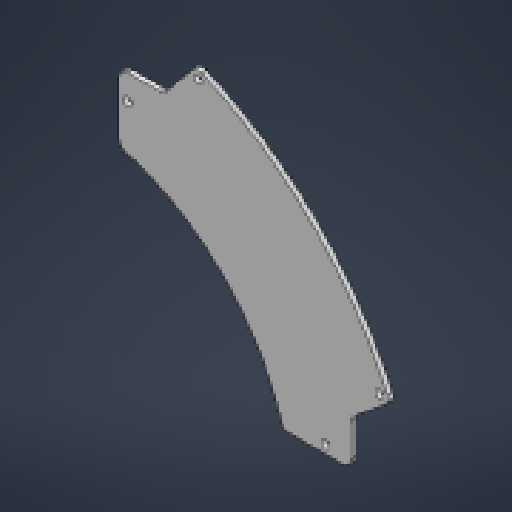
# Autodesk Inventor part: MotorDriver_PCB
Saved by Autodesk Inventor 2024.2 (Build 282272000, 272)
## iProperties
Created: 2023-12-22
Part Number: MotorDriver_PCB
Material: 一般
Document SubType Name: Modeling
Designer: Hanaoka
Density: 1 g/cm^3
Appearance: 既定
Author: Hanaoka
Autodesk Inventor part; units mm, degrees
ref_plane "YZ Plane" through (0, 0, 0) normal (1, 0, 0) x (0, 1, 0)
ref_plane "XZ Plane" through (0, 0, 0) normal (0, 1, 0) x (-1, 0, 0)
ref_plane "XY Plane" through (0, 0, 0) normal (0, 0, 1) x (1, 0, 0)
sketch "スケッチ1" plane through (0, 0, 0) normal (0, 0, 1) x (1, 0, 0)
  line L0 (54, -47.9205) -> (54, -40.1498) projected
  arc A0 (54.7258, -38.6082) -> (54, -40.1498) centre (56, -40.1498) ccw projected
  line L1 (54.7258, -38.6082) -> (62.3004, -32.3475) projected
  arc A1 (62.3004, -32.3475) -> (62.8611, -30.0103) centre (61.0262, -30.8059) ccw projected
  arc A2 (62.8611, -30.0103) -> (17.9102, 14.9406) centre (-16.5, -64.4205) ccw projected
  arc A3 (17.9102, 14.9406) -> (15.573, 14.3799) centre (17.1146, 13.1057) ccw projected
  line L2 (15.573, 14.3799) -> (9.3123, 6.8053) projected
  arc A4 (7.7707, 6.0795) -> (9.3123, 6.8053) centre (7.7707, 8.0795) ccw projected
  line L3 (7.7707, 6.0795) -> (0, 6.0795) projected
  arc A5 (0, 6.0795) -> (-2, 4.0795) centre (0, 4.0795) ccw projected
  line L4 (-2, 4.0795) -> (-2, -8.817) projected
  arc A6 (-2, -8.817) -> (-0.569, -10.7343) centre (0, -8.817) ccw projected
  arc A7 (37.1861, -48.4895) -> (-0.569, -10.7343) centre (-16.5, -64.4205) ccw projected
  arc A8 (37.1861, -48.4895) -> (39.1035, -49.9205) centre (39.1035, -47.9205) ccw projected
  line L5 (39.1035, -49.9205) -> (52, -49.9205) projected
  arc A9 (52, -49.9205) -> (54, -47.9205) centre (52, -47.9205) ccw projected
  circle A10 centre (47.9205, -47.9205) radius 1 projected
  circle A11 centre (0, 0) radius 1 projected
  circle A12 centre (17.1146, 13.1057) radius 1 projected
  circle A13 centre (61.0262, -30.8059) radius 1 projected
  point P0 (0, 0)
extrude "押し出し1" add sketch "スケッチ1" along normal blind 1.2
